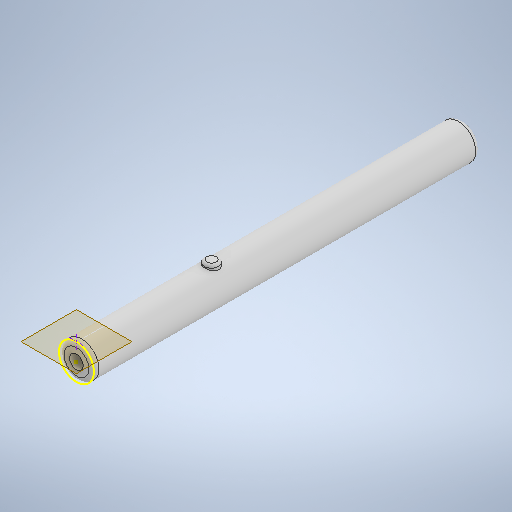
# Autodesk Inventor part: Pen_Model
Saved by Autodesk Inventor 2025 (Build 290162000, 162)
## iProperties
Created: 2024-05-23
Part Number: Pen_Model
Material: Generic
Document SubType Name: Modeling
Designer: mumin
Density: 1 g/cm^3
Appearance: Default
Author: mumin
Autodesk Inventor part; units mm, degrees
ref_plane "YZ Plane" through (0, 0, 0) normal (1, 0, 0) x (0, 1, 0)
ref_plane "XZ Plane" through (0, 0, 0) normal (0, 1, 0) x (-1, 0, 0)
ref_plane "XY Plane" through (0, 0, 0) normal (0, 0, 1) x (1, 0, 0)
sketch "Sketch1" plane through (0, 0, 0) normal (0, 0, 1) x (1, 0, 0)
  circle A0 centre (0, 0) radius 6.925
  dimension "d0" = 13.85
  constraints: 1 centre point, 1 coincident
  measures "d0" diameter of A0
extrude "Extrusion1" add sketch "Sketch1" along normal mid plane 153.5
sketch "Sketch2" plane through (0, 0, 76.75) normal (0, 0, 1) x (1, 0, 0)
  circle A0 centre (0, 0) radius 6.925 projected
  point P0 (0, 6.925)
  constraints: 1 vertical alignment, 1 other
ref_plane "Work Plane1" through (0, 6.925, 76.75) normal (0, 1, 0) x (-1, 0, 0)
sketch "Sketch3" plane through (0, 6.925, 76.75) normal (0, 1, 0) x (-1, 0, 0)
  circle A0 centre (0, -53.585) radius 2.875
  line L0 (6.925, 0) -> (-6.925, 0) projected
  point P0 (0, -76.75)
  dimension "d3" = 50.71
  dimension "d4" = 5.75
  constraints: 1 centre point
  measures "d3" distance edge to line of A0 L0
  measures "d4" diameter of A0
extrude "Extrusion2" add sketch "Sketch3" along normal mid plane 2.92
fillet "Fillet1" radius 1 1 edges at (2.875, 8.385, 23.165)
sketch "Sketch4" plane through (0, 0, 76.75) normal (0, 0, 1) x (1, 0, 0)
  circle A0 centre (0, 0) radius 2.75
  dimension "d8" = 5.5
  constraints: 1 centre point, 1 coincident
  measures "d8" diameter of A0
extrude "Extrusion3" cut sketch "Sketch4" against normal blind 30
fillet "Fillet2" radius 2 2 edges at (-6.925, 0, 76.75) (-6.925, 0, -76.75)
body "Solid1"
